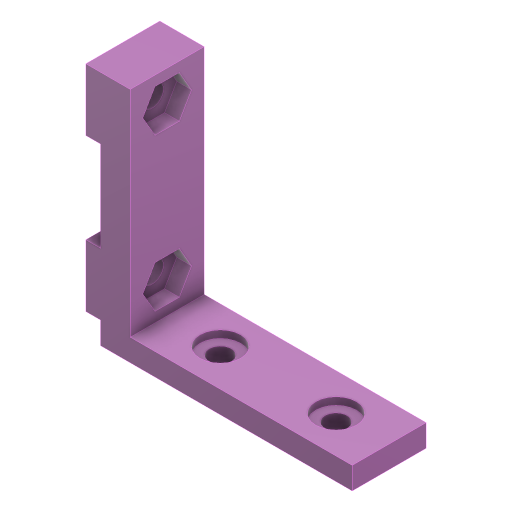
# Autodesk Inventor part: Деталь1
Saved by Autodesk Inventor 2023 (Build 270158000, 158)
## iProperties
Created: 2022-11-25
Part Number: Деталь1
Material: Типовые
Document SubType Name: Modeling
Designer: Admin
Density: 1 g/cm^3
Appearance: По умолчанию
Author: Admin
Autodesk Inventor part; units mm, degrees
ref_plane "YZ Plane" through (0, 0, 0) normal (1, 0, 0) x (0, 1, 0)
ref_plane "XZ Plane" through (0, 0, 0) normal (0, 1, 0) x (-1, 0, 0)
ref_plane "XY Plane" through (0, 0, 0) normal (0, 0, 1) x (1, 0, 0)
sketch "Эскиз1" plane through (0, 0, 0) normal (0, 1, 0) x (-1, 0, 0)
  line L0 (15, 5) -> (-15, 5)
  line L1 (-15, 5) -> (-15, -5)
  line L2 (-15, -5) -> (15, -5)
  line L3 (15, -5) -> (15, 5)
  line L4 (15, 5) -> (-15, -5) construction
  line L5 (-15, 5) -> (15, -5) construction
  line L6 (15, -5) -> (19, -5)
  line L7 (19, -5) -> (19, 5)
  line L8 (19, 5) -> (15, 5)
  line L9 (15, 5) -> (15, -5)
  line L10 (9.4123, -2.75) -> (6.2369, -2.75) construction
  line L11 (6.2369, -2.75) -> (4.6491, 0) construction
  line L12 (4.6491, 0) -> (6.2369, 2.75) construction
  line L13 (6.2369, 2.75) -> (9.4123, 2.75) construction
  line L14 (9.4123, 2.75) -> (11, 0) construction
  line L15 (11, 0) -> (9.4123, -2.75) construction
  line L16 (-6.2369, -2.75) -> (-9.4123, -2.75) construction
  line L17 (-9.4123, -2.75) -> (-11, 0) construction
  line L18 (-11, 0) -> (-9.4123, 2.75) construction
  line L19 (-9.4123, 2.75) -> (-6.2369, 2.75) construction
  line L20 (-6.2369, 2.75) -> (-4.6491, 0) construction
  line L21 (-4.6491, 0) -> (-6.2369, -2.75) construction
  line L22 (0, 0) -> (0, -1.9613) construction
  circle A0 centre (7.8246, 0) radius 2.8 construction
  circle A1 centre (-7.8246, 0) radius 2.8 construction
  circle A2 centre (-7.8246, 0) radius 1.5
  circle A3 centre (7.8246, 0) radius 1.5
  dimension "d0" = 4
  dimension "d1" = 30
  dimension "d2" = 5.6
  dimension "d3" = 5.5
  dimension "d4" = 4
  dimension "d5" = 10
  dimension "d6" = 3
  dimension "d7" = 3
  constraints: 46 end point, 4 centre point, 4 coincident, 4 horizontal, 4 parallel, 3 midpoint, 2 horizontal alignment, 2 perpendicular, 1 collinear, 1 equal radius, 1 symmetric about line, 1 vertical, 26 other
  measures "d0" distance of L2.end L6.end
  measures "d1" distance of L1.end L2.end
  measures "d2" diameter of A0
  measures "d3" distance between parallel lines of L19 L16
  measures "d4" distance from line of L1 L17.end
  measures "d5" distance of L0.end L1.end
  measures "d6" diameter of A3
  measures "d7" diameter of A2
extrude "Выдавливание1" add sketch "Эскиз1" along normal blind 3 contours L3 L2 L1 L0
extrude "Выдавливание2" add sketch "Эскиз1" along normal blind 32 contours L8 L7 L6 L3
sketch "Эскиз2" plane through (-19, 0, -5) normal (-1, 0, 0) x (0, 0, 1)
  circle A0 centre (5, 7.2) radius 1.5
  circle A1 centre (5, 27.8) radius 1.5
  line L0 (0, 0) -> (10, 0) projected
  line L1 (0, 32) -> (10, 32) projected
  line L2 (0, 0) -> (0, 32) projected
  point P0 (5, 0)
  point P1 (5, 32)
  point P2 (5, 0)
  point P3 (0, 3)
  dimension "d13" = 3
  dimension "d14" = 3
  dimension "d17" = 20.6
  dimension "d25" = 4.2
  constraints: 2 centre point, 2 midpoint, 2 vertical alignment
  measures "d13" diameter of A0
  measures "d14" diameter of A1
  measures "d17" distance of A1.centre A0.centre
  measures "d25" vertical distance of point (0, 3) A0.centre
extrude "Выдавливание3" cut sketch "Эскиз2" against normal through all
sketch "Эскиз3" plane through (0, 3, 0) normal (0, 1, 0) x (1, 0, 0)
  circle A0 centre (-7.8246, 0) radius 2.75
  circle A1 centre (7.8246, 0) radius 2.75
  point P0 (0, 0)
  dimension "d20" = 5.5
  dimension "d21" = 5.5
  constraints: 2 centre point, 2 coincident
  measures "d20" diameter of A0
  measures "d21" diameter of A1
extrude "Выдавливание4" cut sketch "Эскиз3" against normal blind 1
sketch "Эскиз4" plane through (-15, 3, -5) normal (1, 0, 0) x (0, 0, -1)
  circle A0 centre (-5, 24.8) radius 1.5 projected
  circle A1 centre (-5, 4.2) radius 1.5 projected
  circle A2 centre (-5, 4.2) radius 1.5 projected
  line L0 (-8.2909, 4.2) -> (-6.6454, 7.05)
  line L1 (-6.6454, 7.05) -> (-3.3546, 7.05)
  line L2 (-3.3546, 7.05) -> (-1.7091, 4.2)
  line L3 (-1.7091, 4.2) -> (-3.3546, 1.35)
  line L4 (-3.3546, 1.35) -> (-6.6454, 1.35)
  line L5 (-6.6454, 1.35) -> (-8.2909, 4.2)
  line L6 (-8.2909, 24.8) -> (-6.6454, 27.65)
  line L7 (-6.6454, 27.65) -> (-3.3546, 27.65)
  line L8 (-3.3546, 27.65) -> (-1.7091, 24.8)
  line L9 (-1.7091, 24.8) -> (-3.3546, 21.95)
  line L10 (-3.3546, 21.95) -> (-6.6454, 21.95)
  line L11 (-6.6454, 21.95) -> (-8.2909, 24.8)
  point P0 (-5, -3)
  dimension "d24" = 5.7
  constraints: 24 end point, 2 coincident, 2 horizontal, 1 parallel, 26 other
  measures "d24" distance between parallel lines of L10 L7
extrude "Выдавливание5" cut sketch "Эскиз4" against normal blind 2
sketch "Эскиз5" plane through (-19, 0, -5) normal (-1, 0, 0) x (0, 0, 1)
  line L0 (0, 3) -> (0, 32) projected
  line L1 (0, 11.4) -> (10, 11.4)
  line L2 (10, 11.4) -> (10, 3)
  line L3 (10, 3) -> (0, 3)
  line L4 (0, 3) -> (0, 11.4)
  line L5 (10, 3) -> (10, 32) projected
  line L6 (0, 32) -> (10, 32)
  line L7 (10, 32) -> (10, 23.6)
  line L8 (10, 23.6) -> (0, 23.6)
  line L9 (0, 23.6) -> (0, 32)
  line L10 (10, 0) -> (10, 32) projected
  circle A0 centre (5, 27.8) radius 1.5 projected
  circle A1 centre (5, 7.2) radius 1.5 projected
  point P0 (5, 0)
  point P1 (10, 27.8)
  point P2 (10, 7.2)
  dimension "d29" = 8.4
  constraints: 16 end point, 4 parallel, 4 point on line, 2 horizontal, 2 horizontal alignment, 2 midpoint, 2 perpendicular
  measures "d29" distance between parallel lines of L3 L1
extrude "Выдавливание6" add sketch "Эскиз5" along normal blind 2 contours L0 L1 L2 L3 | L0 L6 L5 L8
